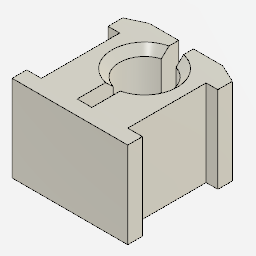
Peg (Autodesk Fusion 360 design; units mm, degrees)
Autodesk Fusion 360 part; units mm, degrees
sketch "Sketch1" plane through (0, 0, 0) normal (0, 0, 1) x (1, 0, 0)
  line L0 (0, 1.75) -> (0, 22.5) construction
  line L1 (1.75, 0) -> (22.5, 0) construction
  line L2 (0, -3.08) -> (-3.16, -3.08)
  line L3 (-3.16, -3.08) -> (-3.16, -2.28)
  line L4 (-3.16, -2.28) -> (-2.36, -2.28)
  line L5 (-2.36, -2.28) -> (-2.36, 2)
  line L6 (-2.36, 2) -> (-3, 2)
  line L7 (-3, 2) -> (-3, 2.8004)
  line L8 (-3, 2.8004) -> (-2, 3.2667)
  line L9 (-2, 3.2667) -> (-0.4, 3.2667)
  line L10 (-0.4, 3.2667) -> (-0.4, -0.3155)
  line L11 (0, -1) -> (0, -2) construction
  line L12 (0.4, 3.2667) -> (0.4, -0.3155)
  line L13 (2, 3.2667) -> (0.4, 3.2667)
  line L14 (3, 2.8004) -> (2, 3.2667)
  line L15 (3, 2) -> (3, 2.8004)
  line L16 (2.36, 2) -> (3, 2)
  line L17 (2.36, -2.28) -> (2.36, 2)
  line L18 (3.16, -2.28) -> (2.36, -2.28)
  line L19 (3.16, -3.08) -> (3.16, -2.28)
  line L20 (0, -3.08) -> (3.16, -3.08)
  line L21 (-0.4, -0.3155) -> (-0.4, -2.28)
  line L22 (-0.4, -2.28) -> (0.4, -2.28)
  line L23 (0.4, -2.28) -> (0.4, 2.3155)
  circle A0 centre (0, 1) radius 1.375
  circle A1 centre (0, 1) radius 1.775
  dimension "d13" = 4.28
  dimension "d14" = 0.8
  dimension "d15" = 0.8
  dimension "d16" = 2.36
  dimension "d17" = 2
  dimension "d18" = 0.16
  dimension "d20" = 1.2667
  dimension "d23" = 115
  dimension "d24" = 1
  dimension "d25" = 0.4
  dimension "d26" = 2.75
  dimension "d27" = 0.4
  dimension "d28" = 0.4
  dimension "d29" = 0.8
  dimension "d45" = 1
  dimension "d47" = 0.4
  constraint horizontal L2
  constraint perpendicular L2 L3
  constraint perpendicular L3 L4
  constraint perpendicular L4 L5
  constraint perpendicular L5 L6
  constraint perpendicular L4 L7
  constraint perpendicular L7 L9
  constraint coincident L0 origin
  constraint perpendicular L9 L10
  constraint vertical L11
  constraint vertical L21
  constraint perpendicular L11 L22
  constraint perpendicular L22 L23
  constraint coincident A0
  constraint coincident origin A0
  constraint concentric A0 A1
  measures "d13" distance of origin
  measures "d14" distance of L3 L5
  measures "d16" distance of L0 L5
  measures "d17" distance of L1 L6
  measures "d18" distance of L3 L7
  measures "d20" distance of L6 L9
  measures "d23" angle of L7 L8
  measures "d24" distance of L7
  measures "d25" distance of L0
  measures "d26" diameter of A0
  measures "d27" distance of L0 L21
  measures "d28" distance of L0 L23
  measures "d29" distance of L20 L22
  measures "d47" distance of A0 A1
extrude "Extrude1" add sketch "Sketch1" against normal blind 4.72 contours L2 L3 L4 L5 L6 L7 L8 L9 L10 L12 L13 L14 L15 L16 L17 L18 L19 L20 L21 L22 L23 A1 | L10 L21 A0 A1 | L12 L23 A0 A1
split_face "SplitFace2" 1 faces at (-1.0533, -1.7631, 0) by curves path "Sketch1" along A1
move_face "OffsetFaces2" offset -0.4 2 faces at (-0.4842, -0.5652, 0) (0.4842, -0.5652, 0)
chamfer "Chamfer1" distance 0.4 angle 45 2 edges at (-1.775, 1, -0.4) (1.775, 1, -0.4)
equation "sheetTh = 4 mm" comment "thickness of the sheet material"
equation "minWallTh = 0.8 mm" comment "minimal thickness of a 3d printed wall"
equation "screewDiam = 3 mm" comment "diameter of the screew"
equation "screewInset = 0.25 mm" comment "inset for the screew"
equation "pegW = 5 mm" comment "width of the peg"
equation "pegOverlap = 0.8 mm" comment "overlapp of the pegs top"
equation "pegOvInset = 0.16 mm" comment "inset between top and bottom peg overlap"
equation "d13 = sheetTh + offsetS"
equation "d14 = pegOverlap"
equation "d15 = minWallTh"
equation "d16 = ( pegW - offsetS ) / 2"
equation "d17 = sheetTh / 2"
equation "d18 = pegOvInset"
equation "d20 = pegEndH + peglengthOffset"
equation "pegSlid = 0.8 mm" comment "slid width inside of the peg"
equation "d25 = pegSlid / 2"
equation "d26 = screewDiam - screewInset"
equation "d27 = pegSlid / 2"
equation "d28 = pegSlid / 2"
equation "d29 = minWallTh"
equation "pegH = pegW"
equation "d31 = -( pegH - offsetS )"
equation "bla = screewDiam + 2 * minWallTh"
equation "offsetW = 0.6 mm"
equation "offsetS = 0.28 mm"
equation "offsetP = 0.18 mm"
equation "screewOffset = 1 mm" comment "off-center of the screew"
equation "d45 = screewOffset"
equation "counterSinkOffset = 0.4 mm"
equation "d47 = counterSinkOffset"
equation "d48 = -counterSinkOffset"
equation "d49 = counterSinkOffset"
equation "screewTheta = minWallTh" comment "minimal distance from counter sink to end of peg"
equation "peglengthOffset = sign(screewOffset - screewTheta) * ( screewOffset - screewTheta )"
equation "pegEndH = minWallTh + minWallTh / 3"
equation "hurga = ( d13 + d15 + pegEndH ) / 2 - screewOffset - ( screewDiam / 2 ) - counterSinkOffset"
